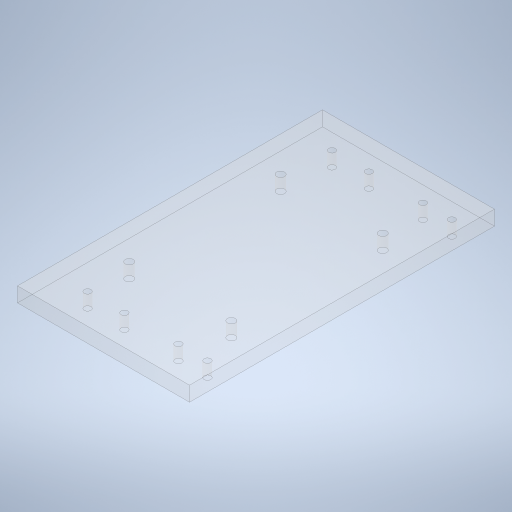
# Autodesk Inventor part: frame_head1
Saved by Autodesk Inventor 2024 (Build 280153000, 153)
## iProperties
Created: 2024-09-08
Part Number: frame_head1
Material: PMMA 플라스틱
Document SubType Name: Modeling
Designer: jmha0
Density: 1.188 g/cm^3
Appearance: 폴리카보네이트 - 선명
Author: jmha0
Autodesk Inventor part; units mm, degrees
ref_plane "YZ Plane" through (0, 0, 0) normal (1, 0, 0) x (0, 1, 0)
ref_plane "XZ Plane" through (0, 0, 0) normal (0, 1, 0) x (-1, 0, 0)
ref_plane "XY Plane" through (0, 0, 0) normal (0, 0, 1) x (1, 0, 0)
sketch "스케치1" plane through (0, 0, 0) normal (0, 1, 0) x (-1, 0, 0)
  circle A0 centre (-8.6694, 43.889) radius 1.35
  circle A1 centre (13.325, 43.8987) radius 1.35
  line L0 (16.8976, 56.1595) -> (-15.4524, 56.1595)
  line L1 (-15.4524, 56.1595) -> (-15.4524, 31.5595)
  line L2 (-15.4524, 31.5595) -> (16.8976, 31.5595)
  line L3 (16.8976, 31.5595) -> (16.8976, 56.1595)
  circle A2 centre (-8.6694, -55.611) radius 1.35
  circle A3 centre (13.325, -55.6013) radius 1.35
  line L4 (16.8976, -43.3405) -> (-15.4524, -43.3405)
  line L5 (-15.4524, -43.3405) -> (-15.4524, -67.9405)
  line L6 (-15.4524, -67.9405) -> (16.8976, -67.9405)
  line L7 (16.8976, -67.9405) -> (16.8976, -43.3405)
  line L8 (-15.4524, 56.1595) -> (44.5476, 56.1595)
  line L9 (44.5476, 56.1595) -> (44.5476, -67.9405)
  line L10 (44.5476, -67.9405) -> (-15.4524, -67.9405)
  line L11 (-15.4524, -67.9405) -> (-15.4524, 56.1595)
  line L12 (-15.4524, 56.1595) -> (-25.4524, 56.1595)
  line L13 (-25.4524, 56.1595) -> (-25.4524, -67.9405)
  line L14 (-25.4524, -67.9405) -> (-15.4524, -67.9405)
  line L15 (-15.4524, -67.9405) -> (-15.4524, 56.1595)
  line L16 (13.325, -55.6013) -> (28.325, -55.6013)
  circle A4 centre (28.325, -55.6013) radius 1.35
  circle A5 centre (28.325, 43.8595) radius 1.35
  circle A6 centre (-20.4524, -55.6013) radius 1.35
  circle A7 centre (-20.4524, 43.8595) radius 1.35
  point P0 (0, 0)
  point P1 (0.7226, 43.8595)
  point P2 (16.8976, -67.9405)
  dimension "d0" = 60
  dimension "d3" = 10
  dimension "d4" = 15
  dimension "d5" = 2.7
  dimension "d6" = 2.7
  dimension "d13" = 2.7
  dimension "d14" = 2.7
  constraints: 34 end point, 8 centre point, 4 parallel, 3 horizontal, 2 perpendicular, 1 coincident, 1 point on line
  measures "d0" distance of L9.end L10.end
  measures "d3" distance of L14.end L13.end
  measures "d4" distance of L16.start L16.end
  measures "d5" diameter of A4
  measures "d6" diameter of A5
  measures "d13" diameter of A6
  measures "d14" diameter of A7
extrude "돌출1" add sketch "스케치1" along normal blind 6
sketch "스케치3" plane through (0, 6, 0) normal (0, 1, 0) x (1, 0, 0)
  line L0 (15.4524, 40.8905) -> (15.4524, -29.1095)
  line L1 (-34.5476, 40.8905) -> (15.4524, 40.8905)
  line L2 (-34.5476, -29.1095) -> (-34.5476, 40.8905)
  line L3 (15.4524, -29.1095) -> (-34.5476, -29.1095)
  line L4 (-44.5476, 67.9405) -> (-44.5476, -56.1595) projected
  line L5 (-44.5476, -56.1595) -> (25.4524, -56.1595) projected
  line L6 (25.4524, -56.1595) -> (25.4524, 67.9405) projected
  line L7 (25.4524, 67.9405) -> (-44.5476, 67.9405) projected
  circle A0 centre (-28.325, 55.6013) radius 1.35 projected
  circle A1 centre (-28.325, -43.8595) radius 1.35 projected
  circle A2 centre (8.6694, 55.611) radius 1.35 projected
  circle A3 centre (20.4524, -43.8595) radius 1.35 projected
  circle A4 centre (20.4524, 55.6013) radius 1.35 projected
  circle A5 centre (-13.325, 55.6013) radius 1.35 projected
  circle A6 centre (-13.325, -43.8987) radius 1.35 projected
  circle A7 centre (8.6694, -43.889) radius 1.35 projected
  circle A8 centre (11.2524, -24.9095) radius 1.6
  circle A9 centre (-30.3476, -24.9095) radius 1.6
  circle A10 centre (-30.3476, 36.6905) radius 1.6
  circle A11 centre (11.2524, 36.6905) radius 1.6
  point P0 (0, 0)
  dimension "d15" = 3.2
  dimension "d16" = 3.2
  dimension "d17" = 3.2
  dimension "d18" = 3.2
  constraints: 8 end point, 4 centre point
  measures "d15" diameter of A8
  measures "d16" diameter of A9
  measures "d17" diameter of A10
  measures "d18" diameter of A11
extrude "돌출2" cut sketch "스케치3" against normal blind 10 contours A8 | A9 | A10 | A11
